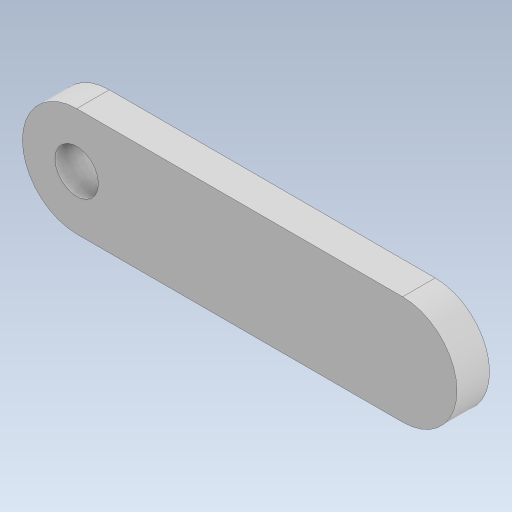
# Autodesk Inventor part: 零件15
Saved by Autodesk Inventor 2023 (Build 270158000, 158)
## iProperties
Created: 2023-06-07
Part Number: 零件15
Material: 一般
Document SubType Name: Modeling
Designer: JOU
Density: 1 g/cm^3
Appearance: 預設
Author: JOU
Autodesk Inventor part; units mm, degrees
ref_plane "YZ Plane" through (0, 0, 0) normal (1, 0, 0) x (0, 1, 0)
ref_plane "XZ Plane" through (0, 0, 0) normal (0, 1, 0) x (-1, 0, 0)
ref_plane "XY Plane" through (0, 0, 0) normal (0, 0, 1) x (1, 0, 0)
sketch "草圖1" plane through (0, 0, 0) normal (0, 0, 1) x (1, 0, 0)
  arc A0 (-220, 5) -> (-220, -5) centre (-220, 0) ccw
  circle A1 centre (-220, 0) radius 2.1
  circle A2 centre (-220, 0) radius 2.1
  line L0 (-220, 0) -> (-190, 0) construction
  line L1 (-220, -5) -> (-190, -5)
  line L2 (-190, 5) -> (-220, 5)
  arc A3 (-220, 5) -> (-220, -5) centre (-220, 0) ccw
  arc A4 (-190, -5) -> (-190, 5) centre (-190, 0) ccw
  line L3 (0, 0) -> (30, 0) construction
  line L4 (0, -5) -> (30, -5)
  line L5 (30, 5) -> (0, 5)
  arc A5 (0, 5) -> (0, -5) centre (0, 0) ccw
  arc A6 (30, -5) -> (30, 5) centre (30, 0) ccw
  circle A7 centre (0, 0) radius 2
  point P0 (-205, 0)
  point P1 (15, 0)
  dimension "d0" = 30
  dimension "d1" = 30
  dimension "d2" = 10
  dimension "d3" = 4
  constraints: 16 end point, 10 point on circle, 8 centre point, 8 tangent, 2 horizontal, 2 midpoint, 2 parallel, 1 coincident
  measures "d0" distance of L0.start L0.end
  measures "d1" distance of L3.start L3.end
  measures "d2" diameter of A6
  measures "d3" diameter of A7
extrude "擠出1" add sketch "草圖1" along normal blind 3 contours A5 L5 A6 L4
